x_idler (Autodesk Fusion 360 design; units mm, degrees)
Autodesk Fusion 360 part; units mm, degrees
note: some values were not read from the file. Set by a fixed rule: which sketch regions a step uses.
sketch "Sketch1" plane through (0, 0, 0) normal (0, 1, 0) x (1, 0, 0)
  circle A0 centre (11, -22.5) radius 5.1
  circle A1 centre (28, -22.5) radius 7.6
  line L0 (0, 0) -> (0, -22.5)
  line L1 (39.5, 0) -> (39.5, -22.5)
  line L2 (39.5, 0) -> (0, 0)
  line L3 (0, -17) -> (16.5, -17)
  arc A2 (16.5, -22.5) -> (39.5, -22.5) centre (28, -22.5) ccw
  arc A3 (0, -22.5) -> (19.1691, -29.8665) centre (11, -22.5) ccw
  line L4 (16.5, -17) -> (16.5, -22.5)
  circle A4 centre (3, -22.5) radius 2
  circle A5 centre (11, -14.5) radius 2
  circle A6 centre (11, -30.5) radius 2
  dimension "d1" = 15.2
  dimension "d2" = 23
  dimension "d3" = 10.2
  dimension "d4" = 22
  dimension "d5" = 17
  dimension "d6" = 22.5
  dimension "d7" = 17
  dimension "d8" = 16
  dimension "d9" = 8
  dimension "d10" = 8
  dimension "d11" = 4
  constraint concentric A0 A3
  constraint concentric A1 A2
  constraint horizontal A1.centre A0.centre
  constraint coincident L0.start L2.end
  constraint tangent L0 A3
  constraint tangent L1 A2
  constraint horizontal L2
  constraint vertical L0
  constraint vertical L1
  constraint coincident L0 L3.start
  constraint perpendicular L1 L3
  constraint coincident A2 A3.end
  constraint tangent A2 L4
  constraint vertical L4
  constraint vertical A0.centre A6.centre
  constraint vertical A0.centre A5.centre
  constraint horizontal A0.centre A4.centre
  constraint equal A4 A5
  constraint equal A4 A6
  measures "d1" diameter of A1
  measures "d2" diameter of A2
  measures "d3" diameter of A0
  measures "d4" diameter of A3
  measures "d5" distance of A0.centre A1.centre
  measures "d6" distance of A0.centre L2
  measures "d7" distance of L2 L3
  measures "d8" distance of A5.centre A6.centre
  measures "d9" distance of A0.centre A6.centre
  measures "d10" distance of A0.centre A4.centre
  measures "d11" diameter of A5
extrude "Extrude1" add sketch "Sketch1" against normal blind 60 contours L0 L1 L2 L3 A2 L4 | A5
extrude "Extrude2" cut sketch "Sketch1" against normal blind 10 contours A5
extrude "Extrude3" add sketch "Sketch1" against normal blind 9 contours L0 L3 A2 A3 L4
sketch "Sketch2" plane through (39.5, 0, 0) normal (1, 0, 0) x (0, 0, -1)
  line L0 (0, 0) -> (-22.5, 0)
  line L1 (-22.5, 0) -> (-22.5, -60)
  line L2 (-22.5, -60) -> (0, -60)
  line L3 (0, -60) -> (0, 0)
  line L4 (-3.75, -15) -> (-13.25, -15)
  line L5 (-13.25, -15) -> (-13.25, -45)
  line L6 (-13.25, -45) -> (-3.75, -45)
  line L7 (-3.75, -45) -> (-3.75, -15)
  line L8 (-3.75, -15) -> (-13.25, -45) construction
  line L9 (-13.25, -15) -> (-3.75, -45) construction
  circle A0 centre (-8.5, -7.5) radius 4.05
  circle A1 centre (-8.5, -52.5) radius 4.05
  point P0 (-8.5, -30)
  dimension "d18" = 8.1
  dimension "d19" = 8.5
  dimension "d20" = 30
  dimension "d21" = 30
  dimension "d22" = 9.5
  dimension "d23" = 45
  dimension "d24" = 22.5
  constraint horizontal L4
  constraint perpendicular L4 L5
  constraint parallel L4 L6
  constraint parallel L5 L7
  constraint coincident L8 P0
  constraint coincident L9 P0
  constraint equal A0 A1
  constraint vertical P0 A0.centre
  constraint vertical A0.centre A1.centre
  measures "d18" diameter of A0
  measures "d19" distance of L3 A0.centre
  measures "d20" distance of L0 P0
  measures "d21" distance of L4.start L6.end
  measures "d22" distance of L4.start L4.end
  measures "d23" distance of A0.centre A1.centre
  measures "d24" distance of P0 A1.centre
extrude "Extrude4" cut sketch "Sketch2" against normal through all contours L4 L5 L6 L7 | A0 | A1
sketch "Sketch3" plane through (0, 0, 17) normal (0, 0, 1) x (1, 0, 0)
  line L0 (16.5, -9) -> (0, -9)
  line L1 (0, -9) -> (0, -60) construction
  line L2 (0, -60) -> (16.5, -60)
  line L3 (16.5, -60) -> (16.5, -9)
  line L4 (0, -15) -> (0, -45)
  circle A0 centre (1.5, -30) radius 15 construction
  line L5 (0, -15) -> (7.7132, -15)
  line L6 (7.7132, -15) -> (16.5, -23.7868)
  line L7 (16.5, -36.2132) -> (7.7132, -45)
  line L8 (7.7132, -45) -> (0, -45)
  point P0 (0, -30)
  dimension "d26" = 30
  dimension "d27" = 45
  dimension "d28" = 45
  constraint midpoint L4 P0
  constraint horizontal A0.centre P0
  constraint tangent L3 A0
  constraint coincident L1 L4.start
  constraint perpendicular L1 L5
  constraint coincident L3 L6.end
  constraint coincident L3 L7.start
  constraint coincident L1 L4.end
  constraint perpendicular L1 L8
  constraint vertical L5.end L7.end
  constraint tangent A0 L7
  constraint tangent A0 L8
  constraint tangent A0 L5
  measures "d26" diameter of A0
  measures "d27" angle of L7 L8
  measures "d28" angle of L5 L6
extrude "Extrude5" cut sketch "Sketch3" against normal through all
fillet "Fillet1" radius 3 5 edges at (0, -12, 17) (0, -52.5, 17) (0, -52.5, 0) (0, -7.5, 0) (19.1691, -4.5, 29.8665)
sketch "Sketch4" plane through (0, 0, 0) normal (0, 1, 0) x (-1, 0, 0)
  arc A0 (-3, 0) -> (0, 3) centre (-3, 3) ccw
  line L0 (0, 3) -> (0, 22.5)
  arc A1 (0, 22.5) -> (-17.3493, 31.4826) centre (-11, 22.5) ccw
  arc A2 (-20.9262, 31.5671) -> (-39.5, 22.5) centre (-28, 22.5) ccw
  line L1 (-39.5, 22.5) -> (-39.5, 0)
  line L2 (-39.5, 0) -> (-3, 0)
  circle A3 centre (-11, 30.5) radius 2
  circle A4 centre (-3, 22.5) radius 2
  circle A5 centre (-11, 22.5) radius 5.1
  circle A6 centre (-11, 14.5) radius 2
  circle A7 centre (-28, 22.5) radius 7.6
  line L3 (-35.6, 22.5) -> (-39.5, 22.5)
  line L4 (-35.5339, 23.5) -> (-39.4564, 23.5)
  arc A8 (-20.9262, 31.5671) -> (-17.3493, 31.4826) centre (-19.0809, 33.9324) ccw
  dimension "d32" = 1
  constraint coincident A7 L3.start
  constraint coincident L1 A2.end
  constraint perpendicular L1 L3
  constraint coincident A7 L4.start
  constraint coincident A2 L4.end
  constraint horizontal L4
  constraint horizontal A2.centre L3.start
  measures "d32" distance of L3 L4
extrude "Extrude6" cut sketch "Sketch4" against normal through all contours A2 A7 L3 L4
sketch "Sketch5" plane through (0, -10, 0) normal (0, 1, 0) x (-1, 0, 0)
  circle A0 centre (-11, 14.5) radius 2
  circle A1 centre (-11, 14.5) radius 1.75
  dimension "d34" = 3.5
  constraint concentric A0 A1
  measures "d34" diameter of A1
extrude "Extrude7" add sketch "Sketch5" along normal blind 5
sketch "Sketch6" plane through (0, 0, 0) normal (0, 0, 1) x (1, 0, 0)
  circle A0 centre (27.9782, -40) radius 2.5
  circle A1 centre (27.9782, -40) radius 6.75
  line L0 (36.9782, -36.2721) -> (31.7061, -31)
  line L1 (31.7061, -31) -> (24.2503, -31)
  line L2 (24.2503, -31) -> (18.9782, -36.2721)
  line L3 (18.9782, -36.2721) -> (18.9782, -43.7279)
  line L4 (18.9782, -43.7279) -> (24.2503, -49)
  line L5 (24.2503, -49) -> (31.7061, -49)
  line L6 (31.7061, -49) -> (36.9782, -43.7279)
  line L7 (36.9782, -43.7279) -> (36.9782, -36.2721)
  line L8 (27.9782, -40) -> (27.9782, -49) construction
  line L9 (27.9782, -40) -> (25.3951, -46.2362)
  line L10 (27.9782, -40) -> (30.5613, -46.2362)
  line L11 (27.9782, -40) -> (21.6143, -46.364) construction
  line L12 (22.4981, -47.2478) -> (24.5891, -45.8375)
  line L13 (20.7304, -45.4801) -> (22.1407, -43.3891)
  line L14 (33.4583, -47.2478) -> (31.3674, -45.8375)
  line L15 (35.2261, -45.4801) -> (33.8157, -43.3891)
  line L16 (36.9782, -41.25) -> (34.5024, -41.7312)
  line L17 (36.9782, -38.75) -> (34.5024, -38.2688)
  line L18 (35.2261, -34.5199) -> (33.8157, -36.6109)
  line L19 (33.4583, -32.7522) -> (31.3674, -34.1625)
  line L20 (29.2282, -31) -> (29.7095, -33.4758)
  line L21 (26.7282, -31) -> (26.247, -33.4758)
  line L22 (22.4981, -32.7522) -> (24.5891, -34.1625)
  line L23 (20.7304, -34.5199) -> (22.1407, -36.6109)
  line L24 (18.9782, -38.75) -> (21.454, -38.2688)
  line L25 (18.9782, -41.25) -> (21.454, -41.7312)
  line L26 (16.5, -60) -> (39.4564, -60)
  point P0 (27.9782, -40)
  point P1 (27.9782, -60)
  dimension "d37" = 5
  dimension "d38" = 13.5
  dimension "d39" = 18
  dimension "d40" = 45
  dimension "d41" = 22.5
  dimension "d42" = 2.5
  dimension "d43" = 1.25
  dimension "d44" = 11
  dimension "d45" = 11
  dimension "d47" = 360
  dimension "d48" = 20
  constraint concentric A0 A1
  constraint coincident P0 A0.centre
  constraint midpoint L5 L8.end
  constraint coincident A1 L9.end
  constraint coincident A1 L10.end
  constraint vertical L8
  constraint vertical L7
  constraint midpoint L4 L11.end
  constraint coincident L4 L12.start
  constraint coincident A1 L12.end
  constraint coincident L4 L13.start
  constraint coincident A1 L13.end
  constraint midpoint L26 P1
  constraint vertical P0 P1
  measures "d37" diameter of A0
  measures "d38" diameter of A1
  measures "d39" distance of L3 L7
  measures "d40" angle of L9 L10
  measures "d41" angle of L8 L9
  measures "d42" distance of L12.start L13.start
  measures "d43" distance of L11.end L13.start
  measures "d44" angle of L11 L12
  measures "d45" angle of L11 L13
  measures "d48" distance of P0 P1
emboss "Emboss1" depth -0.5 profiles "Sketch6" section 1 contours A0 A1 L9 L10 | A1 L4 L12 L13 | A1 L6 L14 L15 | A1 L3 L24 L25 | A1 L7 L16 L17 | A1 L2 L22 L23 | A1 L0 L18 L19 | A1 L1 L20 L21 picked at (32.4003, -42.9646) onto face at (22.5566, -40, 32.6301)
sketch "Sketch7" plane through (0, -60, 0) normal (0, -1, 0) x (1, 0, 0)
  line L0 (39.5, 22.5) -> (35.6, 22.5)
  arc A0 (35.5339, 23.5) -> (35.6, 22.5) centre (28, 22.5) ccw
  line L1 (35.5339, 23.5) -> (39.4564, 23.5)
  arc A1 (39.4564, 23.5) -> (16.5, 22.5) centre (28, 22.5) ccw
  line L2 (16.5, 22.5) -> (16.5, 17)
  line L3 (16.5, 17) -> (3, 17)
  arc A2 (3, 17) -> (0, 14) centre (3, 14) ccw
  line L4 (0, 14) -> (0, 3)
  arc A3 (0, 3) -> (3, 0) centre (3, 3) ccw
  line L5 (3, 0) -> (39.5, 0)
  line L6 (39.5, 0) -> (39.5, 22.5)
  line L7 (22.4165, 23.4975) -> (22.4165, 20.4975)
  line L8 (22.4165, 23.4975) -> (19.4208, 26.4989)
  line L9 (19.4208, 26.4989) -> (19.4123, 17.4989)
  line L10 (19.4123, 17.4989) -> (22.4165, 20.4975)
  point P0 (20.4165, 21.9989)
  point P1 (19.4165, 21.9989)
  dimension "d54" = 2
  dimension "d56" = 45
  dimension "d57" = 45
  dimension "d58" = 3
  dimension "d59" = 1
  dimension "d60" = 9
  constraint vertical L7
  constraint midpoint A0 P0
  constraint horizontal P0 P1
  constraint midpoint P1 L9
  measures "d54" distance of L7 P0
  measures "d56" angle of L8 L9
  measures "d57" angle of L9 L10
  measures "d58" distance of L7.start L7.end
  measures "d59" distance of P0 P1
  measures "d60" vertical distance of L8.end L9.end
extrude "Extrude8" add sketch "Sketch7" against normal blind 11 contours A0 L7 L8 L10
equation "d9 = d8 / 2"
equation "d10 = d9"
equation "d19 = ( 17 / 2 ) * 1 mm"
equation "d24 = d23 / 2"
equation "d28 = d27"
equation "d38 = d37 * 2.7"
equation "d39 = d37 * 3.6"
equation "d40 = ( 360 / 8 ) * 1 deg"
equation "d41 = d40 / 2"
equation "d42 = d37 / 2"
equation "d43 = d42 / 2"
equation "d45 = d44"
equation "d57 = d56"
